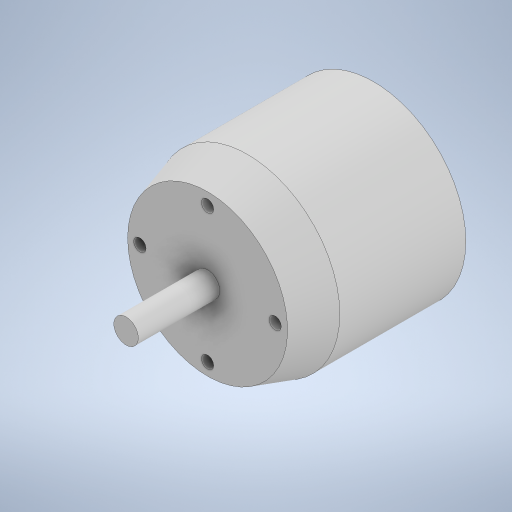
# Autodesk Inventor part: CH-1-02-driveMotor
Saved by Autodesk Inventor 2023 (Build 270158000, 158)
## iProperties
Created: 2022-12-14
Part Number: CH-1-02-driveMotor
Material: Generic
Document SubType Name: Modeling
Designer: megan
Density: 1 g/cm^3
Appearance: Default
Author: megan
Autodesk Inventor part; units mm, degrees
ref_plane "YZ Plane" through (0, 0, 0) normal (1, 0, 0) x (0, 1, 0)
ref_plane "XZ Plane" through (0, 0, 0) normal (0, 1, 0) x (-1, 0, 0)
sketch "Sketch1" plane through (0, 0, 0) normal (0, 0, 1) x (1, 0, 0)
  circle A0 centre (0, 0) radius 30
  dimension "d0" = 60
  constraints: 1 centre point, 1 coincident
  measures "d0" diameter of A0
extrude "Extrusion1" add sketch "Sketch1" along normal blind 41
ref_plane "Work Plane1" through (0, 0, 54) normal (0, 0, 1) x (1, 0, 0)
sketch "Sketch2" plane through (0, 0, 54) normal (0, 0, 1) x (1, 0, 0)
  circle A0 centre (0, 0) radius 26
  dimension "d4" = 52
  constraints: 1 centre point, 1 coincident
  measures "d4" diameter of A0
loft "Loft1" add profiles "Sketch2" section 1 edges at (-30, 0, 41)
sketch "Sketch4" plane through (0, 0, 54) normal (0, 0, 1) x (1, 0, 0)
  point P0 (0, 0)
sketch "Sketch5" plane through (0, 0, 54) normal (0, 0, 1) x (1, 0, 0)
  circle A0 centre (0, 22) radius 2
  circle A1 centre (0, -22) radius 2
  circle A2 centre (0, 0) radius 22
  circle A3 centre (-22, 0) radius 2
  circle A4 centre (22, 0) radius 2
  dimension "d11" = 4
  dimension "d12" = 44
  constraints: 5 centre point, 4 point on circle, 3 equal radius, 1 coincident
  measures "d11" diameter of A0
  measures "d12" diameter of A2
extrude "Extrusion2" cut sketch "Sketch5" against normal blind 5 contours A0 A2 | A2 A0 | A3 A2 | A2 A3 | A4 A2 | A2 A4 | A2 A1 | A1 A2
sketch "Sketch6" plane through (0, 0, 0) normal (0, 0, -1) x (-1, 0, 0)
  point P0 (0, 0)
sketch "Sketch7" plane through (0, 0, 54) normal (0, 0, 1) x (1, 0, 0)
  circle A0 centre (0, 0) radius 4
  dimension "d16" = 8
  constraints: 1 centre point, 1 coincident
  measures "d16" diameter of A0
extrude "Extrusion3" add sketch "Sketch7" along normal blind 26.5 and the other way blind 58
body "Solid1"
